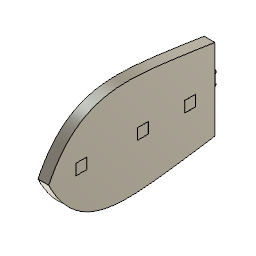
dress_petal (Autodesk Fusion 360 design; units mm, degrees)
part number: 2025-10-09-12-26-06-301
Autodesk Fusion 360 part; units mm, degrees
note: some values were not read from the file. Set by a fixed rule: which sketch regions a step uses.
sketch "Sketch1" plane through (0, 0, 0) normal (0, 0, 1) x (1, 0, 0)
  circle A0 centre (0, 0) radius 1.5
  circle A1 centre (0, 0) radius 3.5
  line L0 (-1.5, 0) -> (1.5, 0)
  line L1 (1.5, 0) -> (1.5, -80)
  line L2 (1.5, -80) -> (-1.5, -80)
  line L3 (-1.5, -80) -> (-1.5, 0)
  line L4 (-20, 0) -> (26, 0) construction
  line L5 (1.5, -14) -> (7.5, -14)
  line L6 (7.5, -14) -> (7.5, -20)
  line L7 (7.5, -20) -> (1.5, -20)
  line L8 (1.5, -20) -> (1.5, -14)
  line L9 (1.5, -40) -> (7.5, -40)
  line L10 (7.5, -40) -> (7.5, -46)
  line L11 (7.5, -46) -> (1.5, -46)
  line L12 (1.5, -46) -> (1.5, -40)
  line L13 (1.5, -80) -> (7.5, -80)
  line L14 (7.5, -80) -> (7.5, -74)
  line L15 (7.5, -74) -> (1.5, -74)
  line L16 (1.5, -74) -> (1.5, -80)
  dimension "d4" = 3
  dimension "d5" = 2
  dimension "d6" = 80
  dimension "d7" = 6
  dimension "d8" = 6
  dimension "d9" = 6
  dimension "d10" = 6
  dimension "d11" = 6
  dimension "d12" = 6
  dimension "d13" = 3
  dimension "d14" = 20
  constraint coincident A0.centre A1.centre
  constraint horizontal L0
  constraint vertical L1
  constraint horizontal L2
  constraint vertical L3
  constraint coincident A0 L0.end
  constraint coincident A0 L0.start
  constraint perpendicular L1 L4
  constraint horizontal L5
  constraint vertical L6
  constraint horizontal L7
  constraint vertical L8
  constraint coincident L1 L5.start
  constraint horizontal L9
  constraint vertical L10
  constraint horizontal L11
  constraint vertical L12
  constraint midpoint L1 L9.start
  constraint horizontal L13
  constraint vertical L14
  constraint horizontal L15
  constraint vertical L16
  measures "d4" diameter of A0
  measures "d5" distance of A0 A1
  measures "d6" distance of L0.start L2.end
  measures "d7" distance of L5.start L7.end
  measures "d8" distance of L5.start L5.end
  measures "d9" distance of L9.start L11.end
  measures "d10" distance of L9.start L9.end
  measures "d11" distance of L14.end L15.end
  measures "d12" distance of L13.end L14.end
  measures "d13" distance of L0.start L0.end
  measures "d14" distance of L7 L9
extrude "Extrude1" add sketch "Sketch1" along normal blind 6 contours A0 A1 L1 L3 | A0 A1 L1 L3 | A1 L1 L2 L3 L8 L12 L16 | L1 L5 L6 L7 L8 | L1 L13 L14 L15 L16 | L1 L9 L10 L11 L12 makes body 1
sketch "Sketch2" plane through (0, 0, 0) normal (1, 0, 0) x (0, 1, 0)
  spline S0 degree 5 poles (-95, 0) (-94.2581, 1.5147) (-92.7272, 4.4413) (-90.2899, 8.5232) (-86.7563, 13.345) (-81.858, 18.317) (-76.4757, 22.2184) (-70.6218, 25.0576) (-64.335, 26.8869) (-57.6941, 27.8301) (-50.8037, 28.0563) (-43.778, 27.753) (-36.726, 27.1016) (-29.7377, 26.2557) (-22.8683, 25.3162) (-16.1468, 24.3428) (-10.8972, 23.5607) (-7.0323, 22.9764) (-4.4876, 22.5879) (-3.2232, 22.394) knots 0 0 0 0 0 0 0.066667 0.133333 0.2 0.266667 0.333333 0.4 0.466667 0.533333 0.6 0.666667 0.733333 0.8 0.866667 0.933333 1 1 1 1 1 1
  line L0 (-3.2232, 0) -> (-3.2232, 22.394)
  line L1 (-80, 3) -> (-74, 3)
  line L2 (-74, 3) -> (-74, -3)
  line L3 (-74, -3) -> (-80, -3)
  line L4 (-80, -3) -> (-80, 3)
  line L5 (-46.0416, 2.9858) -> (-40.0416, 2.9858)
  line L6 (-40.0416, 2.9858) -> (-40.0416, -3.0142)
  line L7 (-40.0416, -3.0142) -> (-46.0416, -3.0142)
  line L8 (-46.0416, -3.0142) -> (-46.0416, 2.9858)
  line L9 (-19.9942, 2.9654) -> (-13.9942, 2.9654)
  line L10 (-13.9942, 2.9654) -> (-13.9942, -3.0346)
  line L11 (-13.9942, -3.0346) -> (-19.9942, -3.0346)
  line L12 (-19.9942, -3.0346) -> (-19.9942, 2.9654)
  line L13 (-80, 3) -> (-74, -3) construction
  line L14 (-74, 3) -> (-80, -3) construction
  line L15 (-46.0416, 2.9858) -> (-40.0416, -3.0142) construction
  line L16 (-40.0416, 2.9858) -> (-46.0416, -3.0142) construction
  line L17 (-19.9942, 2.9654) -> (-13.9942, -3.0346) construction
  line L18 (-13.9942, 2.9654) -> (-19.9942, -3.0346) construction
  line L19 (-3.1623, 0) -> (-14, 0) construction
  spline S1 degree 5 poles (-95, 0) (-94.2581, -1.5147) (-92.7272, -4.4413) (-90.2899, -8.5232) (-86.7563, -13.345) (-81.858, -18.317) (-76.4757, -22.2184) (-70.6218, -25.0576) (-64.335, -26.8869) (-57.6941, -27.8301) (-50.8037, -28.0563) (-43.778, -27.753) (-36.726, -27.1016) (-29.7377, -26.2557) (-22.8683, -25.3162) (-16.1468, -24.3428) (-10.8972, -23.5607) (-7.0323, -22.9764) (-4.4876, -22.5879) (-3.2232, -22.394) knots 0 0 0 0 0 0 0.066667 0.133333 0.2 0.266667 0.333333 0.4 0.466667 0.533333 0.6 0.666667 0.733333 0.8 0.866667 0.933333 1 1 1 1 1 1
  line L20 (-100.5407, -11.3111) -> (-89.4593, 11.3111)
  line L21 (-13.189, 23.9228) -> (6.7426, 20.8651)
  line L22 (-100.5407, 11.3111) -> (-89.4593, -11.3111)
  line L23 (-13.189, -23.9228) -> (6.7426, -20.8651)
  line L24 (-3.2232, 0) -> (-3.2232, -22.394)
  point P0 (-70, 25)
  point P1 (-36.4082, 27.0172)
  point P2 (-70, -25)
  point P3 (-36.4082, -27.0172)
  dimension "d17" = 6
  dimension "d18" = 6
  dimension "d19" = 6
  dimension "d20" = 6
  dimension "d21" = 6
  dimension "d22" = 6
  constraint vertical L0
  constraint horizontal L1
  constraint vertical L2
  constraint horizontal L3
  constraint vertical L4
  constraint horizontal L5
  constraint vertical L6
  constraint horizontal L7
  constraint vertical L8
  constraint horizontal L9
  constraint vertical L10
  constraint horizontal L11
  constraint vertical L12
  constraint midpoint S0.start L20
  constraint midpoint S0.end L21
  constraint symmetric S0.start L19 S1.start
  constraint symmetric P0 L19 P2
  constraint symmetric P1 L19 P3
  constraint symmetric L0.start L19 L24.start
  constraint symmetric S0.end L19 S1.end
  constraint symmetric L19 L20.start L22.start
  constraint symmetric L19 L20.end L22.end
  constraint symmetric L19 L21.start L23.start
  constraint symmetric L19 L21.end L23.end
  measures "d17" distance of L1.start L3.end
  measures "d18" distance of L2.end L3.end
  measures "d19" distance of L5.start L5.end
  measures "d20" distance of L5.start L7.end
  measures "d21" distance of L9.start L11.end
  measures "d22" distance of L10.end L11.end
extrude "Extrude2" add sketch "Sketch2" along normal blind 6 separate body makes body 2
move_body "Move1" bodies 2 to x (1, 0, 0) y (0, 1, 0) z (0, 0, 1) at (0, 0, 3)
move_body "Move2" bodies 2 to x (1, 0, 0) y (0, 1, 0) z (0, 0, 1) at (1.5, 0, 0)
equation "hole_diam = 3 mm"
equation "hole_dist = 2 mm"
equation "petal_len = 40 mm"
equation "d4 = hole_diam"
equation "d5 = hole_dist"
